Autodesk Fusion 360 part; units mm, degrees
note: some values were not read from the file. Set by a fixed rule: which sketch regions a step uses.
(part 2 of 2)
  arc A42 (-31, -9) -> (-30, -8) centre (-31, -8) ccw
  line L390 (-30, -8) -> (-30, 32.9032)
  point P0 (-64.904, -21)
  dimension "d83" = 5
  dimension "d86" = 20
  dimension "d87" = 11.5
  dimension "d88" = 5
  dimension "d89" = 3
  dimension "d91" = 4
  constraint coincident L20.start L21.start
  constraint midpoint L19 L20.end
  constraint midpoint L346 L382.start
  constraint perpendicular L305 L382
  constraint tangent A8 A35
  constraint coincident A34 A35.end
  constraint coincident A8 A35.end
  constraint tangent L382 A36
  constraint tangent A35 A36
  constraint perpendicular L365 L383
  constraint symmetric L382.start L383 L384.start
  constraint symmetric A35.end L383 A37.start
  constraint symmetric A35 L383 A37
  constraint symmetric L382.end L383 L384.end
  constraint symmetric A35.start L383 A37.end
  constraint symmetric A36 L383 A38
  constraint midpoint A34 L386.end
  constraint midpoint A29 L387.end
  measures "d83" distance of L20.start L19
  measures "d89" radius of A36
extrude "Extrude13" cut sketch "Sketch16" against normal blind 13 contours L31 L32 L374 L388 | L278 L279 L280 A34 L386 | L77 L78 L80 L374 | L44 L45 L46 L47 L388 | L278 A34 L386 | L224 L225 L227 A27 L374 | L127 L128 L129 L130 L131 L374 | L126 L127 L130 L374 | L10 L63 L65 L66 L384 L385 A39 L388 | L10 L144 L145 L378 L384 L385 L388 | L63 L64 L65 L385 A39 | L145 L378 L385 | A8 L299 L303 L304 A41 | L199 L200 L201 L202 L203 L374 | L152 L153 L155 L374 | L10 L87 L88 L89 L90 L384 L385 L388 | L10 L114 L115 L116 L117 L384 L385 L388 | L216 L217 L220 L378 | L168 L169 L170 L172 L173 L378 | L115 L116 L385 | L8 A8 L281 L282 L284 L285 L286 L382 A41 L389 A42 L390 | L88 L89 L385 | L242 L243 L245 L378 | L240 L241 L242 L244 L245 L378 | L8 L343 L347 L378 L382 L390 | L293 L294 L297 L378 | L8 L326 L329 L330 L331 L382 L390 | L8 L305 L308 L309 L310 L382 L390 | L14 L15 L16 L17 L18 L19 L20 L21 | L19 L20 L21 | L57 L58 L59 L60 L61 L62 | L81 L82 L83 L84 L85 L86 | L102 L103 L104 L105 L106 L107 | L108 L109 L110 L111 L112 L113 | L132 L133 L134 L135 L136 L137 | L138 L139 L140 L141 L142 L143 | L156 L157 L158 L159 L160 L161 | L162 L163 L164 L165 L166 L167 | L180 L181 L182 L183 L184 L185 | L186 L187 L188 L189 L190 L191 | L204 L205 L206 L207 L208 L209 | L210 L211 L212 L213 L214 L215 | L228 L229 L230 L231 L232 L233 | L234 L235 L236 L237 L238 L239 | L252 L253 L254 L255 L256 L257 | L258 L259 L260 L261 L262 L263 | L264 L265 L266 L267 L268 L269 | L287 L288 L289 L290 L291 L292 | L311 L312 L313 L314 L315 L316 bodies 6
chamfer "Chamfer3" distance 2.5 angle 45 16 edges at (0, -35.9032, -21) (-71.1144, -33.4136, -21) (-73.604, -5.6173, -21) (-71.1144, 22.1789, -21) (-54.8582, 24.6685, -21) (-43.5614, 25.0983, -21) (-43.0998, 26.8492, -21) (-40.5438, 33.4674, -21) (0, 35.9025, -21) (40.5438, 33.4673, -21) (43.0998, 26.8492, -21) (43.5614, 25.0983, -21) (54.8582, 24.6685, -21) (71.1144, 22.1789, -21) (73.604, -5.6173, -21) (71.1144, -33.4136, -21) on bodies 6
sketch "Sketch18" plane through (0, 0, -8) normal (0, 0, 1) x (-1, 0, 0)
  circle A0 centre (36.0404, 18.4681) radius 3.5
  circle A1 centre (60.5404, -6.0319) radius 3.5
  line L0 (31, -9) -> (32, -9)
  arc A2 (42, -19) -> (32, -9) centre (32, -19) ccw
  line L1 (42, -19) -> (42, -20)
  arc A3 (42, -20) -> (43, -21) centre (43, -20) ccw
  line L2 (43, -21) -> (64.904, -21)
  arc A4 (64.904, -21) -> (70.104, -15.8) centre (64.904, -15.8) ccw
  line L3 (70.104, -15.8) -> (70.104, 27.3)
  arc A5 (70.104, 27.3) -> (64.904, 32.5) centre (64.904, 27.3) ccw
  line L4 (64.904, 32.5) -> (31, 32.5)
  arc A6 (31, 32.5) -> (30, 31.5) centre (31, 31.5) ccw
  line L5 (30, 31.5) -> (30, -8)
  arc A7 (30, -8) -> (31, -9) centre (31, -8) ccw
  circle A8 centre (36.0404, -6.0319) radius 3.5
  circle A9 centre (60.5404, 18.4681) radius 3.5
  line L6 (64.5615, 0.9188) -> (64.5615, 11.0146)
  line L7 (63.4615, 12.1146) -> (55.6615, 12.1146)
  line L8 (54.5615, 13.2146) -> (54.5615, 24.7692)
  line L9 (53.4615, 25.8692) -> (42.3421, 25.8692)
  line L10 (41.2421, 24.7692) -> (41.2421, 13.2146)
  line L11 (40.1421, 12.1146) -> (35.6615, 12.1146)
  line L12 (34.5615, 11.0146) -> (34.5615, 0.9188)
  line L13 (35.6615, -0.1812) -> (40.9205, -0.1812)
  line L14 (63.4615, -0.1812) -> (55.6615, -0.1812)
  line L15 (54.5615, -1.2812) -> (54.5615, -14.0812)
  line L16 (51.1689, -15.1812) -> (53.4615, -15.1812)
  arc A10 (50.0761, -14.2061) -> (41.5212, -0.3597) centre (31.0777, -16.3781) ccw
  arc A11 (53.4615, -15.1812) -> (54.5615, -14.0812) centre (53.4615, -14.0812) ccw
  arc A12 (50.0761, -14.2061) -> (51.1689, -15.1812) centre (51.1689, -14.0812) ccw
  arc A13 (35.6615, 12.1146) -> (34.5615, 11.0146) centre (35.6615, 11.0146) ccw
  arc A14 (34.5615, 0.9188) -> (35.6615, -0.1812) centre (35.6615, 0.9188) ccw
  arc A15 (41.5212, -0.3597) -> (40.9205, -0.1812) centre (40.9205, -1.2812) ccw
  arc A16 (42.3421, 25.8692) -> (41.2421, 24.7692) centre (42.3421, 24.7692) ccw
  arc A17 (40.1421, 12.1146) -> (41.2421, 13.2146) centre (40.1421, 13.2146) ccw
  arc A18 (54.5615, 13.2146) -> (55.6615, 12.1146) centre (55.6615, 13.2146) ccw
  arc A19 (64.5615, 11.0146) -> (63.4615, 12.1146) centre (63.4615, 11.0146) ccw
  arc A20 (55.6615, -0.1812) -> (54.5615, -1.2812) centre (55.6615, -1.2812) ccw
  arc A21 (63.4615, -0.1812) -> (64.5615, 0.9188) centre (63.4615, 0.9188) ccw
  arc A22 (54.5615, 24.7692) -> (53.4615, 25.8692) centre (53.4615, 24.7692) ccw
  line L17 (0, 1) -> (0, 10)
  arc A23 (-41.5212, -0.3597) -> (-50.0761, -14.2061) centre (-31.0777, -16.3781) ccw
  circle A24 centre (-36.0404, -6.0319) radius 3.5
  arc A25 (-35.6615, -0.1812) -> (-34.5615, 0.9188) centre (-35.6615, 0.9188) ccw
  line L18 (-34.5615, 11.0146) -> (-34.5615, 0.9188)
  arc A26 (-34.5615, 11.0146) -> (-35.6615, 12.1146) centre (-35.6615, 11.0146) ccw
  circle A27 centre (-36.0404, 18.4681) radius 3.5
  arc A28 (-32, -9) -> (-42, -19) centre (-32, -19) ccw
  arc A29 (-54.5615, -1.2812) -> (-55.6615, -0.1812) centre (-55.6615, -1.2812) ccw
  line L19 (-40.1421, 12.1146) -> (-35.6615, 12.1146)
  line L20 (-35.6615, -0.1812) -> (-40.9205, -0.1812)
  line L21 (-63.4615, -0.1812) -> (-55.6615, -0.1812)
  line L22 (-64.5615, 0.9188) -> (-64.5615, 11.0146)
  arc A30 (-64.5615, 0.9188) -> (-63.4615, -0.1812) centre (-63.4615, 0.9188) ccw
  arc A31 (-63.4615, 12.1146) -> (-64.5615, 11.0146) centre (-63.4615, 11.0146) ccw
  circle A32 centre (-60.5404, 18.4681) radius 3.5
  arc A33 (-41.2421, 24.7692) -> (-42.3421, 25.8692) centre (-42.3421, 24.7692) ccw
  arc A34 (-40.9205, -0.1812) -> (-41.5212, -0.3597) centre (-40.9205, -1.2812) ccw
  line L23 (-54.5615, 13.2146) -> (-54.5615, 24.7692)
  arc A35 (-55.6615, 12.1146) -> (-54.5615, 13.2146) centre (-55.6615, 13.2146) ccw
  line L24 (-63.4615, 12.1146) -> (-55.6615, 12.1146)
  circle A36 centre (-60.5404, -6.0319) radius 3.5
  line L25 (-31, -9) -> (-32, -9)
  line L26 (-51.1689, -15.1812) -> (-53.4615, -15.1812)
  arc A37 (-51.1689, -15.1812) -> (-50.0761, -14.2061) centre (-51.1689, -14.0812) ccw
  line L27 (-54.5615, -1.2812) -> (-54.5615, -14.0812)
  arc A38 (-54.5615, -14.0812) -> (-53.4615, -15.1812) centre (-53.4615, -14.0812) ccw
  arc A39 (-53.4615, 25.8692) -> (-54.5615, 24.7692) centre (-53.4615, 24.7692) ccw
  line L28 (-41.2421, 24.7692) -> (-41.2421, 13.2146)
  line L29 (-53.4615, 25.8692) -> (-42.3421, 25.8692)
  arc A40 (-41.2421, 13.2146) -> (-40.1421, 12.1146) centre (-40.1421, 13.2146) ccw
  circle A41 centre (-60.5404, -7.0319) radius 2.75
  circle A42 centre (-36.0404, 17.4681) radius 2.75
  circle A43 centre (-60.5404, 17.4681) radius 2.75
  line L30 (-30, -32.9025) -> (-30, 32.9032)
  circle A44 centre (-36.0404, -7.0319) radius 2.75
  line L31 (-30, 32.9032) -> (-65.104, 32.9032)
  arc A45 (-65.104, 32.9032) -> (-70.604, 27.4032) centre (-65.104, 27.4032) ccw
  line L32 (-70.604, 27.4032) -> (-70.604, -16.1685)
  arc A46 (-70.604, -16.1685) -> (-65.104, -21.6685) centre (-65.104, -16.1685) ccw
  line L33 (-65.104, -21.6685) -> (-44.6124, -21.6685)
  arc A47 (-40.1132, -26.0867) -> (-44.6124, -21.6685) centre (-44.6124, -26.1685) ccw
  line L34 (-40.1132, -26.0867) -> (-40.0874, -27.5026)
  arc A48 (-40.0874, -27.5026) -> (-34.5883, -32.9025) centre (-34.5883, -27.4025) ccw
  line L35 (-34.5883, -32.9025) -> (-30, -32.9025)
  point P0 (-64.904, 27.3)
  point P1 (-64.904, -15.8)
  dimension "d99" = 1.1
  constraint parallel L3 L6
  constraint perpendicular L6 L7
  constraint perpendicular L7 L8
  constraint perpendicular L8 L9
  constraint perpendicular L9 L10
  constraint perpendicular L10 L11
  constraint perpendicular L11 L12
  constraint perpendicular L10 L13
  constraint perpendicular L6 L14
  constraint perpendicular L14 L15
  constraint perpendicular L15 L16
  constraint tangent L15 A11
  constraint tangent L16 A11
  constraint tangent A10 A12
  constraint tangent L16 A12
  constraint equal A11 A12
  constraint tangent L11 A13
  constraint tangent L12 A13
  constraint equal A11 A13
  constraint tangent L12 A14
  constraint tangent L13 A14
  constraint equal A11 A14
  constraint tangent L13 A15
  constraint tangent A10 A15
  constraint equal A11 A15
  constraint tangent L9 A16
  constraint tangent L10 A16
  constraint equal A11 A16
  constraint tangent L10 A17
  constraint tangent L11 A17
  constraint equal A11 A17
  constraint tangent L7 A18
  constraint tangent L8 A18
  constraint equal A11 A18
  constraint tangent L6 A19
  constraint tangent L7 A19
  constraint equal A11 A19
  constraint tangent L14 A20
  constraint tangent L15 A20
  constraint equal A11 A20
  constraint tangent L6 A21
  constraint tangent L14 A21
  constraint equal A11 A21
  constraint tangent L8 A22
  constraint tangent L9 A22
  constraint equal A11 A22
  constraint vertical L17
  constraint symmetric A0 L17 A27
  constraint symmetric A1 L17 A36
  constraint symmetric L0.start L17 L25.start
  constraint symmetric L0.end L17 A28.start
  constraint symmetric A2.start L17 A28.end
  constraint symmetric A2 L17 A28
  constraint symmetric A4.centre L17 P1
  constraint symmetric A5.centre L17 P0
  constraint symmetric A8 L17 A24
  constraint symmetric A9 L17 A32
  constraint symmetric A10 L17 A23
  constraint symmetric L15.end L17 L27.end
  constraint symmetric L16.end L17 L26.end
  constraint symmetric A11 L17 A38
  constraint symmetric L16.start L17 L26.start
  constraint symmetric A10.start L17 A23.end
  constraint symmetric A12 L17 A37
  constraint symmetric L11.end L17 A26.end
  constraint symmetric L12.start L17 L18.start
  constraint symmetric A13 L17 A26
  constraint symmetric L12.end L17 A25.end
  constraint symmetric L13.start L17 A25.start
  constraint symmetric A14 L17 A25
  constraint symmetric L13.end L17 L20.end
  constraint symmetric A10.end L17 A23.start
  constraint symmetric A15 L17 A34
  constraint symmetric L9.end L17 A33.end
  constraint symmetric L10.start L17 A33.start
  constraint symmetric A16 L17 A33
  constraint symmetric L10.end L17 L28.end
  constraint symmetric L11.start L17 L19.start
  constraint symmetric A17 L17 A40
  constraint symmetric L7.end L17 A35.start
  constraint symmetric L8.start L17 L23.start
  constraint symmetric A18 L17 A35
  constraint symmetric L6.end L17 L22.end
  constraint symmetric L7.start L17 A31.start
  constraint symmetric A19 L17 A31
  constraint symmetric L14.end L17 A29.end
  constraint symmetric L15.start L17 A29.start
  constraint symmetric A20 L17 A29
  constraint symmetric L6.start L17 L22.start
  constraint symmetric L14.start L17 L21.start
  constraint symmetric A21 L17 A30
  constraint symmetric L8.end L17 L23.end
  constraint symmetric L9.start L17 A39.start
  constraint symmetric A22 L17 A39
  measures "d99" radius of A11
extrude "Extrude14" [suppressed]
sketch "Sketch19" plane through (0, 0, 0) normal (0, 0, 1) x (-1, 0, 0)
  arc A0 (34.5883, -32.9025) -> (40.0874, -27.5026) centre (34.5883, -27.4025) ccw
  line L0 (34.5883, -32.9025) -> (-34.5883, -32.9025)
  arc A1 (-40.0874, -27.5026) -> (-34.5883, -32.9025) centre (-34.5883, -27.4025) ccw
  line L1 (-40.0874, -27.5026) -> (-40.1132, -26.0867)
  arc A2 (-40.1132, -26.0867) -> (-44.6124, -21.6685) centre (-44.6124, -26.1685) ccw
  line L2 (-44.6124, -21.6685) -> (-65.104, -21.6685)
  arc A3 (-70.604, -16.1685) -> (-65.104, -21.6685) centre (-65.104, -16.1685) ccw
  line L3 (-70.604, -16.1685) -> (-70.604, 27.4032)
  arc A4 (-65.104, 32.9032) -> (-70.604, 27.4032) centre (-65.104, 27.4032) ccw
  line L4 (-65.104, 32.9032) -> (65.104, 32.9032)
  arc A5 (70.604, 27.4032) -> (65.104, 32.9032) centre (65.104, 27.4032) ccw
  line L5 (70.604, 27.4032) -> (70.604, -16.1685)
  arc A6 (65.104, -21.6685) -> (70.604, -16.1685) centre (65.104, -16.1685) ccw
  line L6 (65.104, -21.6685) -> (44.6124, -21.6685)
  arc A7 (44.6124, -21.6685) -> (40.1132, -26.0867) centre (44.6124, -26.1685) ccw
  line L7 (40.1132, -26.0867) -> (40.0874, -27.5026)
  circle A8 centre (36.0404, -6.0319) radius 2.75
  circle A9 centre (36.0404, 18.4681) radius 2.75
  circle A10 centre (60.5404, 18.4681) radius 2.75
  circle A11 centre (60.5404, -6.0319) radius 2.75
  circle A12 centre (-36.0404, 17.4681) radius 2.75
  circle A13 centre (-60.5404, 17.4681) radius 2.75
  circle A14 centre (-60.5404, -7.0319) radius 2.75
  line L8 (-47.9307, -16.2852) -> (-64.9552, -16.2852)
  line L9 (-64.9552, -16.2852) -> (-64.9552, -19.4255)
  line L10 (-64.9552, -19.4255) -> (-47.9307, -19.4255)
  line L11 (-47.9307, -19.4255) -> (-47.9307, -16.2852)
  line L12 (-65.104, 32.4032) -> (65.104, 32.4032)
  arc A15 (-65.104, 32.4032) -> (-70.104, 27.4032) centre (-65.104, 27.4032) ccw
  line L13 (-70.104, -16.1685) -> (-70.104, 27.4032)
  arc A16 (-70.104, -16.1685) -> (-65.104, -21.1685) centre (-65.104, -16.1685) ccw
  line L14 (-44.6124, -21.1685) -> (-65.104, -21.1685)
  arc A17 (-39.6132, -26.0776) -> (-44.6124, -21.1685) centre (-44.6124, -26.1685) ccw
  arc A18 (-39.5875, -27.4935) -> (-34.5883, -32.4025) centre (-34.5883, -27.4025) ccw
  line L15 (-39.5875, -27.4935) -> (-39.6132, -26.0776)
  line L16 (34.5883, -32.4025) -> (-34.5883, -32.4025)
  arc A19 (34.5883, -32.4025) -> (39.5875, -27.4935) centre (34.5883, -27.4025) ccw
  arc A20 (44.6124, -21.1685) -> (39.6132, -26.0776) centre (44.6124, -26.1685) ccw
  line L17 (39.5875, -27.4935) -> (39.6132, -26.0776)
  line L18 (44.6124, -21.1685) -> (65.104, -21.1685)
  arc A21 (65.104, -21.1685) -> (70.104, -16.1685) centre (65.104, -16.1685) ccw
  line L19 (70.104, -16.1685) -> (70.104, 27.4032)
  arc A22 (70.104, 27.4032) -> (65.104, 32.4032) centre (65.104, 27.4032) ccw
  line L20 (-40.1897, -14.3954) -> (-56.1897, -14.3954)
  line L21 (-56.1897, -14.3954) -> (-56.1897, 1.6046)
  line L22 (-56.1897, 1.6046) -> (-40.1897, 1.6046)
  line L23 (-40.1897, 1.6046) -> (-40.1897, -14.3954)
  line L24 (-67.2289, -2.0568) -> (-67.2289, 13.9432)
  line L25 (-51.2289, 13.9432) -> (-51.2289, -2.0568)
  line L26 (-67.2289, 13.9432) -> (-51.2289, 13.9432)
  line L27 (-51.2289, -2.0568) -> (-67.2289, -2.0568)
  line L28 (-43.4552, -2.3096) -> (-43.4552, 13.6904)
  line L29 (-27.4552, 13.6904) -> (-27.4552, -2.3096)
  line L30 (-43.4552, 13.6904) -> (-27.4552, 13.6904)
  line L31 (-27.4552, -2.3096) -> (-43.4552, -2.3096)
  line L32 (-56.0936, 12.1136) -> (-56.0936, 28.1136)
  line L33 (-40.0936, 28.1136) -> (-40.0936, 12.1136)
  line L34 (-56.0936, 28.1136) -> (-40.0936, 28.1136)
  line L35 (-40.0936, 12.1136) -> (-56.0936, 12.1136)
  circle A23 centre (-36.0404, -7.0319) radius 2.75
  spline S0 degree 5 poles (-27.4552, -2.3096) (-27.783, -2.3096) (-28.4387, -2.3096) (-29.4223, -2.3096) (-30.7336, -2.3096) (-32.3728, -2.3096) (-33.6842, -2.3096) (-34.6677, -2.3096) (-35.3234, -2.3096) (-35.6513, -2.3096) knots 0 0 0 0 0 0 0.2 0.4 0.6 0.8 1 1 1 1 1 1
  line L36 (-25, -31) -> (-35.6828, -31)
  line L37 (-35.6828, -31) -> (-35.6828, -15)
  line L38 (-35.6828, -15) -> (-25, -15)
  line L39 (-25, -15) -> (-25, -31)
  line L40 (-23.2334, -32.4025) -> (-23.2334, -12.4491)
  line L41 (-24.3334, -11.3491) -> (-25.4, -11.3491)
  line L42 (-27.5, -9.2491) -> (-27.5, 21.5338)
  line L43 (0, 0) -> (0, -11.8761)
  line L44 (-25.4, 23.6338) -> (31.699, 23.6338)
  line L45 (31.699, 23.6338) -> (31.699, 32.4032)
  line L46 (-0.6905, -16.5747) -> (-0.6905, 23.6338)
  line L47 (23.3977, -12.9574) -> (23.3977, 23.6338)
  line L48 (27.4552, 13.6904) -> (27.4552, -0.2096)
  line L49 (29.5552, -2.3096) -> (43.4552, -2.3096)
  line L50 (43.4552, -2.3096) -> (43.4552, 13.6904)
  line L51 (56.1897, 1.6046) -> (40.1897, 1.6046)
  line L52 (40.1897, 1.6046) -> (40.1897, -14.3954)
  line L53 (40.1897, -14.3954) -> (56.1897, -14.3954)
  line L54 (56.1897, -14.3954) -> (56.1897, 1.6046)
  line L55 (40.0936, 12.1136) -> (56.0936, 12.1136)
  line L56 (67.2289, 13.9432) -> (51.2289, 13.9432)
  line L57 (51.2289, 13.9432) -> (51.2289, -2.0568)
  line L58 (51.2289, -2.0568) -> (67.2289, -2.0568)
  line L59 (67.2289, -2.0568) -> (67.2289, 13.9432)
  line L60 (43.4552, 13.6904) -> (27.4552, 13.6904)
  line L61 (40.0936, 28.1136) -> (40.0936, 12.1136)
  line L62 (56.0936, 12.1136) -> (56.0936, 28.1136)
  line L63 (56.0936, 28.1136) -> (40.0936, 28.1136)
  line L64 (41.7132, -15.963) -> (70.104, -15.963)
  line L65 (39.6132, -18.063) -> (39.6132, -26.0776)
  line L66 (23.3977, -16.5747) -> (-0.6905, -16.5747)
  line L67 (23.3977, -32.9025) -> (23.3977, -32.4025)
  line L68 (23.3977, -16.5747) -> (23.3977, -12.9574)
  line L69 (27.4552, 13.6904) -> (27.4552, 23.6338)
  line L70 (31.9131, -2.3096) -> (31.9131, -9.5905)
  line L71 (34.0131, -11.6905) -> (40.1897, -11.6905)
  line L72 (40.1897, -14.3954) -> (40.1897, -15.963)
  line L73 (46.6898, -15.963) -> (46.6898, -21.1685)
  arc A24 (-23.2334, -12.4491) -> (-24.3334, -11.3491) centre (-24.3334, -12.4491) ccw
  arc A25 (31.9131, -9.5905) -> (34.0131, -11.6905) centre (34.0131, -9.5905) ccw
  arc A26 (27.4552, -0.2096) -> (29.5552, -2.3096) centre (29.5552, -0.2096) ccw
  arc A27 (41.7132, -15.963) -> (39.6132, -18.063) centre (41.7132, -18.063) ccw
  arc A28 (-27.5, -9.2491) -> (-25.4, -11.3491) centre (-25.4, -9.2491) ccw
  arc A29 (-25.4, 23.6338) -> (-27.5, 21.5338) centre (-25.4, 21.5338) ccw
  line L74 (39.6132, -26.0776) -> (39.6132, -11.6905)
  arc A30 (-43.0869, -27.5571) -> (-34.5883, -35.9025) centre (-34.5883, -27.4025) ccw
  line L75 (-34.5883, -35.9025) -> (34.5883, -35.9025)
  arc A31 (34.5883, -35.9025) -> (43.0869, -27.5571) centre (34.5883, -27.4025) ccw
  line L76 (43.0869, -27.5571) -> (43.1127, -26.1412)
  arc A32 (44.6124, -24.6685) -> (43.1127, -26.1412) centre (44.6124, -26.1685) ccw
  line L77 (44.6124, -24.6685) -> (65.104, -24.6685)
  arc A33 (65.104, -24.6685) -> (73.604, -16.1685) centre (65.104, -16.1685) ccw
  line L78 (73.604, -16.1685) -> (73.604, 27.4032)
  arc A34 (73.604, 27.4032) -> (65.104, 35.9032) centre (65.104, 27.4032) ccw
  line L79 (65.104, 35.9032) -> (-65.104, 35.9032)
  arc A35 (-65.104, 35.9032) -> (-73.604, 27.4032) centre (-65.104, 27.4032) ccw
  line L80 (-73.604, 27.4032) -> (-73.604, -16.1685)
  arc A36 (-73.604, -16.1685) -> (-65.104, -24.6685) centre (-65.104, -16.1685) ccw
  line L81 (-65.104, -24.6685) -> (-44.6124, -24.6685)
  arc A37 (-43.1127, -26.1412) -> (-44.6124, -24.6685) centre (-44.6124, -26.1685) ccw
  line L82 (-43.1127, -26.1412) -> (-43.0869, -27.5571)
  line L83 (-7.3482, 23.6338) -> (-7.3482, -32.4025)
  line L84 (-18.6213, -32.9025) -> (-18.6213, 23.6338)
  line L85 (40.1897, -14.3954) -> (39.6132, -14.3954)
  line L86 (66.0675, -15.963) -> (66.0675, -21.0748)
  point P0 (-38.7904, -7.0319)
  point P1 (60.5404, 17.4681)
  dimension "d102" = 16
  dimension "d103" = 16
  dimension "d104" = 16
  dimension "d105" = 16
  dimension "d106" = 16
  dimension "d107" = 16
  dimension "d108" = 16
  dimension "d109" = 16
  dimension "d113" = 1.1
  dimension "d114" = 2.1
  constraint horizontal L8
  constraint vertical L9
  constraint horizontal L10
  constraint vertical L11
  constraint horizontal L20
  constraint vertical L21
  constraint horizontal L22
  constraint vertical L23
  constraint horizontal L27
  constraint vertical L24
  constraint horizontal L26
  constraint vertical L25
  constraint horizontal L31
  constraint vertical L28
  constraint horizontal L30
  constraint vertical L29
  constraint horizontal L35
  constraint vertical L32
  constraint horizontal L34
  constraint vertical L33
  constraint coincident L31 S0.end
  constraint horizontal L36
  constraint vertical L37
  constraint horizontal L38
  constraint vertical L39
  constraint coincident L16 L40.start
  constraint perpendicular L38 L40
  constraint perpendicular L40 L41
  constraint perpendicular L12 L42
  constraint coincident L43.start origin
  constraint perpendicular L16 L43
  constraint perpendicular L42 L44
  constraint coincident L12 L45.end
  constraint perpendicular L12 L45
  constraint coincident L44 L46.end
  constraint vertical L46
  constraint coincident L44 L47.end
  constraint perpendicular L44 L47
  constraint coincident L0 L67.start
  constraint perpendicular L16 L67
  constraint symmetric A13.centre L43 P1
  constraint symmetric L20.start L43 L52.end
  constraint symmetric L20.end L43 L53.end
  constraint symmetric L21.end L43 L51.start
  constraint symmetric L22.end L43 L51.end
  constraint symmetric L24.start L43 L58.end
  constraint symmetric L24.end L43 L56.start
  constraint symmetric L25.end L43 L57.end
  constraint symmetric L25.start L43 L56.end
  constraint symmetric L28.start L43 L49.end
  constraint symmetric L28.end L43 L50.end
  constraint symmetric L29.start L43 L48.start
  constraint symmetric L32.start L43 L55.end
  constraint symmetric L32.end L43 L62.end
  constraint symmetric L33.end L43 L55.start
  constraint symmetric L33.start L43 L61.start
  constraint coincident L19 L64.end
  constraint perpendicular L19 L64
  constraint perpendicular L64 L65
  constraint perpendicular L46 L66
  constraint coincident L16 L67.end
  constraint collinear L67 L68
  constraint coincident L66.start L67
  constraint coincident L44 L69.end
  constraint perpendicular L44 L69
  constraint coincident L49 L70.start
  constraint perpendicular L49 L70
  constraint coincident L52 L71.end
  constraint perpendicular L52 L71
  constraint coincident L64 L72.end
  constraint perpendicular L64 L72
  constraint coincident L64 L73.start
  constraint coincident L18 L73.end
  constraint perpendicular L18 L73
  constraint coincident A20.end L17.end
  constraint tangent L40 A24
  constraint tangent L41 A24
  constraint tangent L70 A25
  constraint tangent L71 A25
  constraint tangent L48 A26
  constraint tangent L49 A26
  constraint equal A25 A26
  constraint tangent L64 A27
  constraint tangent L65 A27
  constraint equal A25 A27
  constraint tangent L41 A28
  constraint tangent L42 A28
  constraint equal A25 A28
  constraint tangent L44 A29
  constraint tangent L42 A29
  constraint equal A25 A29
  constraint coincident L71 L74.end
  constraint perpendicular L71 L74
  constraint coincident L44 L83.start
  constraint coincident L16 L83.end
  constraint perpendicular L16 L83
  constraint coincident L0 L84.start
  constraint coincident L44 L84.end
  constraint perpendicular L44 L84
  constraint coincident L74 L85.end
  constraint perpendicular L74 L85
  constraint coincident L64 L86.start
  constraint coincident A21 L86.end
  constraint perpendicular L64 L86
  measures "d102" distance of L20.start L20.end
  measures "d103" distance of L20 L22
  measures "d104" distance of L24.start L25.end
  measures "d105" distance of L26 L27
  measures "d106" distance of L28.start L29.end
  measures "d107" distance of L30 L31
  measures "d108" distance of L32.start L33.end
  measures "d109" distance of L34 L35
  measures "d113" radius of A24
  measures "d114" radius of A25
extrude "Extrude15" add sketch "Sketch19" along normal blind 3 separate body contours L16 L44 L83 L84 | L12 A15 L13 A16 L14 A17 A18 L15 L16 L20 L21 L23 L24 L26 L27 L30 L31 L32 L33 L34 S0 L40 L41 L42 L44 L45 A24 A28 A29 | A20 L18 L64 L65 L73 A27 L74 | L44 L46 L47 L66 L68 | L12 L19 A22 L44 L45 L53 L54 L56 L58 L59 L60 L61 L62 L63 L64 L69 A27 L74 L85 | A21 L19 L64 L86 makes body 9
combine "Combine3" operation add target body 7 tool bodies 8 6
extrude "Extrude16" add 1 faces at (-21.7013, -33.9032, 0) along direction (0, 0, 1) blind 3 on bodies 4 bodies 4
chamfer "Chamfer1" distance 1 angle 45 16 edges at (0, -35.9032, 3) (71.1144, -33.4136, 3) (73.604, -5.6173, 3) (71.1144, 22.1789, 3) (54.8582, 24.6685, 3) (43.5614, 25.0983, 3) (43.0998, 26.8492, 3) (40.5438, 33.4673, 3) (0, 35.9025, 3) (-40.5438, 33.4674, 3) (-43.0998, 26.8492, 3) (-43.5614, 25.0983, 3) (-54.8582, 24.6685, 3) (-71.1144, 22.1789, 3) (-73.604, -5.6173, 3) (-71.1144, -33.4136, 3) on bodies 4
combine "Combine4" operation add target body 4 tool bodies 7
sketch "Sketch20" plane through (0, 35.9025, 0) normal (0, 1, 0) x (-1, 0, 0)
  line L0 (34.5883, 2) -> (-34.5883, 2)
  line L1 (-34.5883, 2) -> (-34.5883, -19)
  line L2 (-34.5883, -19) -> (34.5883, -19)
  line L3 (34.5883, -19) -> (34.5883, 2)
  line L4 (-20.1055, -19) -> (-4.8945, -19)
  line L5 (-4.8945, -19) -> (-4.8945, -16.5)
  line L6 (-4.8945, -16.5) -> (-20.1055, -16.5)
  line L7 (-20.1055, -16.5) -> (-20.1055, -19)
  line L8 (-20.1055, -16.5) -> (-12.5, -11.1745)
  line L9 (-12.5, -11.1745) -> (-4.8945, -16.5)
  line L10 (-20.1055, -18) -> (-4.8945, -18)
  line L11 (34.5883, 2) -> (-34.5883, 2)
  line L12 (-34.5883, 2) -> (-34.5883, -18.5)
  line L13 (-34.5883, -18.5) -> (34.5883, -18.5)
  line L14 (34.5883, -18.5) -> (34.5883, 2)
  line L15 (-34.5883, -21) -> (34.5883, -21)
  line L16 (-20.1055, -19) -> (-20.1055, -21)
  line L17 (-4.8945, -21) -> (-20.1055, -21)
  line L18 (-4.8945, -21) -> (-4.8945, -19)
  dimension "d119" = 35
  dimension "d120" = 35
  dimension "d125" = 3
  dimension "d126" = 1.5
  constraint horizontal L4
  constraint horizontal L6
  constraint coincident L2 L4.start
  constraint coincident L15 L16.end
  constraint perpendicular L15 L16
  constraint coincident L15 L17.start
  constraint perpendicular L4 L18
  measures "d119" angle of L6 L8
  measures "d120" angle of L6 L9
  measures "d125" distance of L10 L17
  measures "d126" distance of L6 L10
extrude "Extrude18" cut sketch "Sketch20" against normal blind 5 contours L5 L6 L7 L10 | L6 L8 L9 bodies 4
hidden bodies 1 2 3 5
equation "d3 = ( 140.208 / 2 ) * 1 mm"
named bodies: "Case Top(test)", "Case Bottom", "Speaker", "Bottom Shell (of bottom)", "CaseTop"
